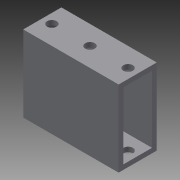
# Autodesk Inventor part: back roller 2x1
Saved by Autodesk Inventor 2015 SP1 (Build 190203100, 203)
## iProperties
Created: 2015-01-25
Part Number: back roller 2x1
Material: Generic
Document SubType Name: Modeling
Designer: Admin
Density: 1 g/cm^3
Appearance: Default
Author: Admin
Autodesk Inventor part; units mm, degrees
ref_plane "YZ Plane" through (0, 0, 0) normal (1, 0, 0) x (0, 1, 0)
ref_plane "XZ Plane" through (0, 0, 0) normal (0, 1, 0) x (-1, 0, 0)
ref_plane "XY Plane" through (0, 0, 0) normal (0, 0, 1) x (1, 0, 0)
sketch "Sketch1" plane through (0, 0, 0) normal (1, 0, 0) x (0, 1, 0)
  line L0 (0, 0) -> (50.8, 0)
  line L1 (50.8, 0) -> (50.8, -25.4)
  line L2 (50.8, -25.4) -> (0, -25.4)
  line L3 (0, -25.4) -> (0, 0)
  line L4 (3.175, -3.175) -> (47.625, -3.175)
  line L5 (47.625, -3.175) -> (47.625, -22.225)
  line L6 (47.625, -22.225) -> (3.175, -22.225)
  line L7 (3.175, -22.225) -> (3.175, -3.175)
  dimension "d0" = 50.8
  dimension "d1" = 25.4
  dimension "d2" = 44.45
  dimension "d3" = 19.05
  dimension "d4" = 3.175
  dimension "d5" = 3.175
  constraints: 16 end point, 4 parallel, 2 horizontal, 2 perpendicular
  measures "d0" distance of L1.end L2.end
  measures "d1" distance of L0.end L1.end
  measures "d2" distance of L5.end L6.end
  measures "d3" distance of L4.end L5.end
  measures "d4" distance between parallel lines of L3 L7
  measures "d5" distance between parallel lines of L0 L4
extrude "Extrusion1" add sketch "Sketch1" along normal blind 63.5
sketch "Sketch2" plane through (0, 50.8, 0) normal (0, 1, 0) x (1, 0, 0)
  line L0 (0, 0) -> (63.5, 0) projected
  line L1 (63.5, 25.4) -> (63.5, 0) projected
  point P0 (57.15, 12.7)
  point P1 (31.75, 12.7)
  point P2 (6.35, 12.7)
  dimension "d8" = 6.35
  dimension "d9" = 31.75
  dimension "d10" = 57.15
  dimension "d11" = 12.7
  dimension "d12" = 12.7
  dimension "d13" = 12.7
  measures "d8" distance from line of point (57.15, 12.7) L1
  measures "d9" distance from line of point (31.75, 12.7) L1
  measures "d10" distance from line of point (6.35, 12.7) L1
  measures "d11" distance from line of L0 point (57.15, 12.7)
  measures "d12" distance from line of L0 point (31.75, 12.7)
  measures "d13" distance from line of L0 point (6.35, 12.7)
hole "Hole1" at (57.15, 50.8, -12.7) at (31.75, 50.8, -12.7) at (6.35, 50.8, -12.7) direction (0, -1, 0) diameter 6.35 end through all
body "Solid1"
